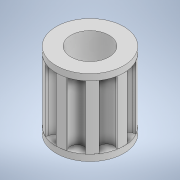
# Autodesk Inventor part: Pièce_moteur_courroie_test_3
Saved by Autodesk Inventor 2020.1 (Build 241239000, 239)
## iProperties
Created: 2019-07-26
Part Number: Pièce_moteur_courroie_test_3
Material: Générique
Document SubType Name: Modeling
Designer: marlo
Density: 1 g/cm^3
Appearance: Par défaut
Author: marlo
Autodesk Inventor part; units mm, degrees
ref_plane "YZ Plane" through (0, 0, 0) normal (1, 0, 0) x (0, 1, 0)
ref_plane "XZ Plane" through (0, 0, 0) normal (0, 1, 0) x (-1, 0, 0)
ref_plane "XY Plane" through (0, 0, 0) normal (0, 0, 1) x (1, 0, 0)
sketch "Esquisse2" plane through (0, 0, 0) normal (0, 1, 0) x (-1, 0, 0)
  circle A0 centre (0, 0) radius 7.975
  dimension "d0" = 15.95
  constraints: 1 centre point, 1 coincident
  measures "d0" diameter of A0
extrude "Extrusion1" add sketch "Esquisse2" along normal blind 15
sketch "Esquisse4" plane through (0, 15, 0) normal (0, 1, 0) x (1, 0, 0)
  circle A0 centre (0, 0) radius 7.975 projected
  circle A1 centre (0, 0) radius 7.975 projected
  arc A2 (-3.2, -7.3048) -> (0, -7.975) centre (0, 0) ccw
  line L0 (-0.0068, -0.0109) -> (-5.0602, -8.1445)
  line L1 (0, -6.3735) -> (0, 5.2233) construction
  line L2 (-3.2, -7.3048) -> (0, -7.975) construction
  line L3 (-3.2, -7.3048) -> (-3.0743, -6.7048)
  line L4 (0, -7.975) -> (0.1257, -7.375)
  arc A3 (0.1257, -7.375) -> (-3.0743, -6.7048) centre (-1.4743, -7.0399) ccw
  line L5 (-3.0743, -6.7048) -> (0.1257, -7.375) construction
  arc A4 (-7.1498, -3.5328) -> (-5.1314, -6.1048) centre (0, 0) ccw
  line L6 (-5.1314, -6.1048) -> (-7.1498, -3.5328) construction
  line L7 (-5.1314, -6.1048) -> (-4.6492, -5.7264)
  line L8 (-7.1498, -3.5328) -> (-6.6676, -3.1544)
  arc A5 (-4.6492, -5.7264) -> (-6.6676, -3.1544) centre (-5.6584, -4.4404) ccw
  line L9 (-4.6492, -5.7264) -> (-6.6676, -3.1544) construction
  line L10 (-5.1314, -6.1048) -> (-3.2, -7.3048) construction
  line L11 (0, 0) -> (-9.6935, -3.168)
  arc A6 (-4.7097, 6.4358) -> (-6.8963, 4.0051) centre (0, 0) ccw
  line L12 (-6.8963, 4.0051) -> (-4.7097, 6.4358) construction
  line L13 (-6.8963, 4.0051) -> (-6.4406, 3.5951)
  line L14 (-4.7097, 6.4358) -> (-4.254, 6.0258)
  arc A7 (-6.4406, 3.5951) -> (-4.254, 6.0258) centre (-5.3473, 4.8105) ccw
  line L15 (-6.4406, 3.5951) -> (-4.254, 6.0258) construction
  arc A8 (-7.7463, 1.8961) -> (-7.8562, -1.3715) centre (0, 0) ccw
  line L16 (-7.7463, 1.8961) -> (-7.8562, -1.3715) construction
  line L17 (-7.7463, 1.8961) -> (-7.1336, 1.8755)
  line L18 (-7.8562, -1.3715) -> (-7.2435, -1.3921)
  arc A9 (-7.2435, -1.3921) -> (-7.1336, 1.8755) centre (-7.1886, 0.2417) ccw
  line L19 (-7.1336, 1.8755) -> (-7.2435, -1.3921) construction
  line L20 (-7.7463, 1.8961) -> (-6.8963, 4.0051) construction
  line L21 (-7.8562, -1.3715) -> (-7.1498, -3.5328) construction
  line L22 (0, 0) -> (-3.9831, 7.4909)
  arc A10 (6.6117, -4.4594) -> (7.8454, -1.4316) centre (0, 0) ccw
  line L23 (7.8454, -1.4316) -> (6.6117, -4.4594) construction
  line L24 (7.8454, -1.4316) -> (7.2777, -1.2003)
  line L25 (6.6117, -4.4594) -> (6.044, -4.228)
  arc A11 (7.2777, -1.2003) -> (6.044, -4.228) centre (6.6609, -2.7142) ccw
  line L26 (7.2777, -1.2003) -> (6.044, -4.228) construction
  arc A12 (7.9306, 0.8406) -> (6.9268, 3.9522) centre (0, 0) ccw
  line L27 (7.9306, 0.8406) -> (6.9268, 3.9522) construction
  line L28 (7.9306, 0.8406) -> (7.3472, 0.6524)
  line L29 (6.9268, 3.9522) -> (6.3434, 3.764)
  arc A13 (6.3434, 3.764) -> (7.3472, 0.6524) centre (6.8453, 2.2082) ccw
  line L30 (7.3472, 0.6524) -> (6.3434, 3.764) construction
  line L31 (7.9306, 0.8406) -> (7.8454, -1.4316) construction
  line L32 (0.5357, 7.957) -> (0.6208, 7.3499)
  arc A14 (-2.617, 6.8962) -> (0.6208, 7.3499) centre (-0.9981, 7.1231) ccw
  line L33 (0.6208, 7.3499) -> (-2.617, 6.8962) construction
  line L34 (0.5357, 7.957) -> (-2.7021, 7.5033) construction
  arc A15 (0.5357, 7.957) -> (-2.7021, 7.5033) centre (0, 0) ccw
  line L35 (-2.7021, 7.5033) -> (-2.617, 6.8962)
  line L36 (2.7595, 7.4824) -> (0.5357, 7.957) construction
  line L37 (2.7595, 7.4824) -> (2.434, 6.9629)
  line L38 (2.434, 6.9629) -> (5.2044, 5.2269) construction
  line L39 (2.7595, 7.4824) -> (5.5299, 5.7463) construction
  arc A16 (5.5299, 5.7463) -> (2.7595, 7.4824) centre (0, 0) ccw
  arc A17 (2.434, 6.9629) -> (5.2044, 5.2269) centre (3.8192, 6.0949) ccw
  line L40 (5.5299, 5.7463) -> (5.2044, 5.2269)
  line L41 (5.5299, 5.7463) -> (6.9268, 3.9522) construction
  line L42 (-4.7097, 6.4358) -> (-2.7021, 7.5033) construction
  line L43 (0, 0) -> (2.483, -17.7205) construction
  arc A18 (2.1919, -7.6679) -> (5.0845, -6.144) centre (0, 0) ccw
  line L44 (5.0845, -6.144) -> (2.1919, -7.6679) construction
  line L45 (5.0845, -6.144) -> (4.7988, -5.6016)
  line L46 (2.1919, -7.6679) -> (1.9062, -7.1255)
  arc A19 (4.7988, -5.6016) -> (1.9062, -7.1255) centre (3.3525, -6.3636) ccw
  line L47 (4.7988, -5.6016) -> (1.9062, -7.1255) construction
  line L48 (6.6117, -4.4594) -> (5.0845, -6.144) construction
  line L49 (2.1919, -7.6679) -> (0, -7.975) construction
  point P0 (-7.7463, 1.8961)
  point P1 (-7.8562, -1.3715)
  point P2 (-4.7097, 6.4358)
  point P3 (0.5357, 7.957)
  point P4 (-2.7021, 7.5033)
  point P5 (5.5299, 5.7463)
  point P6 (2.7595, 7.4824)
  point P7 (7.9306, 0.8406)
  point P8 (6.9268, 3.9522)
  point P9 (6.6117, -4.4594)
  point P10 (7.8454, -1.4316)
  point P11 (-3.2, -7.3048)
  point P12 (0, -7.975)
  point P13 (-7.1498, -3.5328)
  point P14 (-5.1314, -6.1048)
  point P15 (5.0845, -6.144)
  dimension "d14" = 3.2
  dimension "d28" = 0.6
  dimension "d30" = 1.2
  constraints: 100 end point, 41 point on circle, 40 symmetric about line, 18 centre point, 5 point on line, 4 equal length, 3 perpendicular, 1 coincident, 1 midpoint, 1 vertical, 16 other
  measures "d14" horizontal distance of L2.start L2.end
  measures "d28" vertical distance of L2.start L3.end
  measures "d30" vertical distance of L6.start L2.start
extrude "Extrusion6" cut sketch "Esquisse4" against normal blind 15 contours L28 A13 L29 A0 | A0 L25 A11 L24 | L40 A17 L37 A0 | A0 L46 A19 L45 | L32 A14 L35 A0 | A0 L3 A3 L4 | L14 A7 L13 A0 | A0 L8 A5 L7 | L17 A9 L18 A0
sketch "Esquisse6" plane through (0, 15, 0) normal (0, 1, 0) x (1, 0, 0)
  circle A0 centre (0, 0) radius 8
  dimension "d19" = 16
  constraints: 1 centre point, 1 coincident
  measures "d19" diameter of A0
extrude "Extrusion3" add sketch "Esquisse6" along normal blind 1.5
sketch "Esquisse7" plane through (0, 0, 0) normal (0, -1, 0) x (1, 0, 0)
  circle A0 centre (0, 0) radius 8
  constraints: 1 centre point, 1 coincident
extrude "Extrusion4" add sketch "Esquisse7" along normal blind 1.5
sketch "Esquisse8" plane through (0, 16.5, 0) normal (0, 1, 0) x (1, 0, 0)
  circle A0 centre (0, 0) radius 4.5
  dimension "d24" = 9
  constraints: 1 centre point, 1 coincident
  measures "d24" diameter of A0
extrude "Extrusion5" cut sketch "Esquisse8" against normal through all
